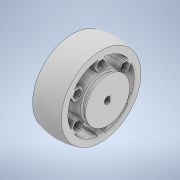
# Autodesk Inventor part: PulleyedWheelV1
Saved by Autodesk Inventor 2020 (Build 240168000, 168)
## iProperties
Created: 2023-12-21
Part Number: PulleyedWheelV1
Material: Generic
Document SubType Name: Modeling
Designer: smz3rm
Density: 1 g/cm^3
Appearance: Default
Author: smz3rm
Autodesk Inventor part; units mm, degrees
ref_plane "YZ Plane" through (0, 0, 0) normal (1, 0, 0) x (0, 1, 0)
ref_plane "XZ Plane" through (0, 0, 0) normal (0, 1, 0) x (-1, 0, 0)
ref_plane "XY Plane" through (0, 0, 0) normal (0, 0, 1) x (1, 0, 0)
sketch "Sketch1" plane through (0, 0, 0) normal (1, 0, 0) x (0, 1, 0)
  circle A0 centre (0, 0) radius 1.5
  line L0 (-25.2, 0) -> (25.2, 0) projected
  line L1 (1.118, -1) -> (-1.118, -1)
  circle A1 centre (0, 0) radius 10
  circle A2 centre (0, 0) radius 18
  circle A3 centre (0, 0) radius 15
  dimension "d0" = 3
  dimension "d1" = 1
  dimension "d3" = 36
  dimension "d4" = 3
  dimension "d6" = 20
  constraints: 4 centre point, 4 coincident, 2 end point, 2 point on circle, 1 horizontal
  measures "d0" diameter of A0
  measures "d1" distance between parallel lines of L0 L1
  measures "d3" diameter of A2
  measures "d4" radial gap between concentric circles of A2 A3
  measures "d6" diameter of A1
extrude "Extrusion1" add sketch "Sketch1" along normal blind 3 contours L1 A0 | A0 L0 A1 | L0 A1 A0
sketch "Sketch3" plane through (0, 0, 0) normal (0, 0, 1) x (1, 0, 0)
  line L0 (0, 10) -> (3, 10) projected
  line L1 (-16.2, 0) -> (6.2, 0) projected
  circle A0 centre (1.5, 9.5) radius 0.5
  line L2 (1.5, 9.5) -> (1.5, 10)
  line L3 (1.067, 9.25) -> (0.634, 10)
  line L4 (0, 10) -> (3, 10) projected
  line L5 (1.933, 9.25) -> (2.366, 10)
  line L6 (0, 10) -> (3, 10) projected
  point P0 (0, 0)
  dimension "d20" = 1
  dimension "d22" = 60
  dimension "d23" = 60
  constraints: 6 end point, 3 tangent, 2 point on circle, 2 point on line, 1 centre point, 1 midpoint, 1 vertical
  measures "d20" diameter of A0
  measures "d22" angle of L0 L3
  measures "d23" angle of L0 L5
revolve "Revolution1" cut sketch "Sketch3" angle 360 about axis through (-10, 0, 0) along (1, 0, 0)
sketch "Sketch2" plane through (0, 0, 0) normal (-1, 0, 0) x (0, 0, 1)
  circle A0 centre (0, 0) radius 18
  circle A1 centre (0, 0) radius 15
  circle A2 centre (0, 0) radius 10 projected
  line L0 (-1, 1.118) -> (-1, -1.118) projected
  arc A3 (-1, -1.118) -> (-1, 1.118) centre (0, 0) ccw projected
  line L1 (1.4537, 14.9294) -> (2.9073, 12.4116)
  line L2 (2.9073, 12.4116) -> (1.4537, 9.8938)
  line L3 (1.4537, 9.8938) -> (-1.4537, 9.8938)
  line L4 (-1.4537, 9.8938) -> (-2.9073, 12.4116)
  line L5 (-2.9073, 12.4116) -> (-1.4537, 14.9294)
  line L6 (-1.4537, 14.9294) -> (1.4537, 14.9294)
  line L7 (0, -25.2) -> (0, 25.2) projected
  line L8 (-0.9918, 14.1294) -> (-1.9836, 12.4116)
  line L9 (-1.9836, 12.4116) -> (-0.9918, 10.6938)
  line L10 (-0.9918, 10.6938) -> (0.9918, 10.6938)
  line L11 (0.9918, 10.6938) -> (1.9836, 12.4116)
  line L12 (1.9836, 12.4116) -> (0.9918, 14.1294)
  line L13 (0.9918, 14.1294) -> (-0.9918, 14.1294)
  line L14 (-12.2024, 3.688) -> (-13.6561, 6.2058)
  line L15 (-9.2951, 3.688) -> (-12.2024, 3.688)
  line L16 (-7.8414, 6.2058) -> (-9.2951, 3.688)
  line L17 (-13.6561, 6.2058) -> (-12.2024, 8.7236)
  line L18 (-12.2024, 8.7236) -> (-9.2951, 8.7236)
  line L19 (-9.2951, 8.7236) -> (-7.8414, 6.2058)
  line L20 (-11.7405, 7.9236) -> (-12.7323, 6.2058)
  line L21 (-12.7323, 6.2058) -> (-11.7405, 4.488)
  line L22 (-11.7405, 4.488) -> (-9.757, 4.488)
  line L23 (-9.757, 4.488) -> (-8.7652, 6.2058)
  line L24 (-8.7652, 6.2058) -> (-9.757, 7.9236)
  line L25 (-9.757, 7.9236) -> (-11.7405, 7.9236)
  line L26 (-9.2951, -8.7236) -> (-12.2024, -8.7236)
  line L27 (-7.8414, -6.2058) -> (-9.2951, -8.7236)
  line L28 (-9.2951, -3.688) -> (-7.8414, -6.2058)
  line L29 (-12.2024, -8.7236) -> (-13.6561, -6.2058)
  line L30 (-13.6561, -6.2058) -> (-12.2024, -3.688)
  line L31 (-12.2024, -3.688) -> (-9.2951, -3.688)
  line L32 (-12.7323, -6.2058) -> (-11.7405, -7.9236)
  line L33 (-11.7405, -7.9236) -> (-9.757, -7.9236)
  line L34 (-9.757, -7.9236) -> (-8.7652, -6.2058)
  line L35 (-8.7652, -6.2058) -> (-9.757, -4.488)
  line L36 (-9.757, -4.488) -> (-11.7405, -4.488)
  line L37 (-11.7405, -4.488) -> (-12.7323, -6.2058)
  line L38 (2.9073, -12.4116) -> (1.4537, -14.9294)
  line L39 (1.4537, -9.8938) -> (2.9073, -12.4116)
  line L40 (-1.4537, -9.8938) -> (1.4537, -9.8938)
  line L41 (1.4537, -14.9294) -> (-1.4537, -14.9294)
  line L42 (-1.4537, -14.9294) -> (-2.9073, -12.4116)
  line L43 (-2.9073, -12.4116) -> (-1.4537, -9.8938)
  line L44 (-0.9918, -14.1294) -> (0.9918, -14.1294)
  line L45 (0.9918, -14.1294) -> (1.9836, -12.4116)
  line L46 (1.9836, -12.4116) -> (0.9918, -10.6938)
  line L47 (0.9918, -10.6938) -> (-0.9918, -10.6938)
  line L48 (-0.9918, -10.6938) -> (-1.9836, -12.4116)
  line L49 (-1.9836, -12.4116) -> (-0.9918, -14.1294)
  line L50 (12.2024, -3.688) -> (13.6561, -6.2058)
  line L51 (9.2951, -3.688) -> (12.2024, -3.688)
  line L52 (7.8414, -6.2058) -> (9.2951, -3.688)
  line L53 (13.6561, -6.2058) -> (12.2024, -8.7236)
  line L54 (12.2024, -8.7236) -> (9.2951, -8.7236)
  line L55 (9.2951, -8.7236) -> (7.8414, -6.2058)
  line L56 (11.7405, -7.9236) -> (12.7323, -6.2058)
  line L57 (12.7323, -6.2058) -> (11.7405, -4.488)
  line L58 (11.7405, -4.488) -> (9.757, -4.488)
  line L59 (9.757, -4.488) -> (8.7652, -6.2058)
  line L60 (8.7652, -6.2058) -> (9.757, -7.9236)
  line L61 (9.757, -7.9236) -> (11.7405, -7.9236)
  line L62 (9.2951, 8.7236) -> (12.2024, 8.7236)
  line L63 (7.8414, 6.2058) -> (9.2951, 8.7236)
  line L64 (9.2951, 3.688) -> (7.8414, 6.2058)
  line L65 (12.2024, 8.7236) -> (13.6561, 6.2058)
  line L66 (13.6561, 6.2058) -> (12.2024, 3.688)
  line L67 (12.2024, 3.688) -> (9.2951, 3.688)
  line L68 (12.7323, 6.2058) -> (11.7405, 7.9236)
  line L69 (11.7405, 7.9236) -> (9.757, 7.9236)
  line L70 (9.757, 7.9236) -> (8.7652, 6.2058)
  line L71 (8.7652, 6.2058) -> (9.757, 4.488)
  line L72 (9.757, 4.488) -> (11.7405, 4.488)
  line L73 (11.7405, 4.488) -> (12.7323, 6.2058)
  point P0 (0, 12.4116)
  point P1 (-1.4537, -14.9294)
  dimension "d9" = 36
  dimension "d10" = 3
  dimension "d11" = 0.8
  dimension "d14" = 360
  constraints: 144 end point, 2 centre point, 2 coincident, 2 point on circle, 1 point on line, 165 other
  measures "d9" diameter of A0
  measures "d10" radial gap between concentric circles of A0 A1
  measures "d11" distance between parallel lines of L5 L8
extrude "Extrusion2" add sketch "Sketch2" along normal blind 13 contours A0 L7 A1 | L7 A1 A0 | L7 L6 A1 | A1 L6 L7 | L7 L41 A1 | A1 L41 L7 | L1 L2 A2 L7 L10 L11 L12 L13 L6 | L6 L7 L13 L8 L9 L10 A2 L4 L5 | L42 L43 A2 L7 L47 L48 L49 L44 L41 | L41 L7 L44 L45 L46 L47 A2 L39 L38 | L65 L66 L67 A2 L63 L62 | A1 L65 | L17 A1 | L18 L19 A2 L15 L14 L17 | L29 L30 L31 A2 L27 L26 | A1 L29 | L53 A1 | L54 L55 A2 L51 L50 L53 | L3 L7 A2 | A2 L64 L52 L40 L7 A3 L3 | L3 L7 A3 L0 L40 A2 L28 L16 | A2 L7 L3 | L40 L7 A2 | A2 L7 L40 | A2 L64 | L16 A2 | A2 L28 | L52 A2
sketch "Sketch4" plane through (0, 0, 0) normal (0, 0, 1) x (1, 0, 0)
  line L0 (0, 18) -> (-13, 18) projected
  line L1 (-13, 18) -> (-13, -18) projected
  arc A0 (0, 18) -> (-13, 18) centre (-6.5, -2.625) ccw
  line L2 (-16.2, 0) -> (6.2, 0) projected
  point P0 (0, 0)
  point P1 (-6.5, 19)
  dimension "d24" = 1
  constraints: 3 point on circle, 1 centre point
  measures "d24" distance from line of L0 point (-6.5, 19)
revolve "Revolution2" add sketch "Sketch4" angle 360 about axis through (-10, 0, 0) along (1, 0, 0)
equation "\"d6\" = WheelGrooveDia"
equation "\"d7\" = WheelGrooveWidth"
equation "\"d20\" = WheelPulleyDia"
equation "\"d9\" = WheelDia - 2 * Roundedness"
equation "\"d16\" = WheelWidth"
equation "\"d24\" = Roundedness"
equation "\"Roundedness\" = 1"
equation "\"WheelGrooveDia\" = 20"
equation "\"WheelGrooveWidth\" = 3"
equation "\"WheelPulleyDia\" = 1"
equation "\"WheelDia\" = 38"
equation "\"WheelWidth\" = 13"
body "Solid1"
